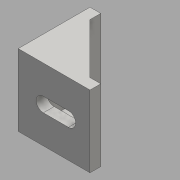
# Autodesk Inventor part: GUSSET 2020
Saved by Autodesk Inventor 2016 (Build 200138000, 138)
## iProperties
Created: 2023-12-31
Part Number: GUSSET 2020
Material: Generic
Document SubType Name: Modeling
Designer: Riskinova Oktavia
Density: 1 g/cm^3
Appearance: Default
Author: Riskinova Oktavia
Autodesk Inventor part; units mm, degrees
ref_plane "YZ Plane" through (0, 0, 0) normal (1, 0, 0) x (0, 1, 0)
ref_plane "XZ Plane" through (0, 0, 0) normal (0, 1, 0) x (-1, 0, 0)
ref_plane "XY Plane" through (0, 0, 0) normal (0, 0, 1) x (1, 0, 0)
sketch "Sketch1" plane through (0, 0, 0) normal (0, 0, 1) x (1, 0, 0)
  line L0 (0, 0) -> (0, 20)
  line L1 (0, 0) -> (20, 0)
  line L2 (0, 20) -> (3, 20)
  line L3 (3, 20) -> (3, 17)
  line L4 (3, 17) -> (17, 3)
  line L5 (17, 3) -> (20, 3)
  line L6 (20, 3) -> (20, 0)
  dimension "d0" = 20
  dimension "d1" = 20
  dimension "d2" = 3
  dimension "d3" = 3
  dimension "d4" = 3
  dimension "d5" = 3
  constraints: 14 end point, 2 horizontal, 2 vertical, 1 parallel, 1 perpendicular
  measures "d0" distance of L0.start L1.end
  measures "d1" distance of L0.start L0.end
  measures "d2" distance of L0.end L2.end
  measures "d3" distance of L5.end L1.end
  measures "d4" distance of L2.end L3.end
  measures "d5" distance of L4.end L5.end
extrude "Extrusion1" add sketch "Sketch1" along normal mid plane 20
sketch "Sketch2" plane through (0, 20, 10) normal (0, 1, 0) x (1, 0, 0)
  line L0 (3, 2) -> (17, 2)
  line L1 (17, 2) -> (17, 18)
  line L2 (17, 18) -> (3, 18)
  line L3 (3, 18) -> (3, 2)
  line L4 (0, 0) -> (0, 20) projected
  line L5 (3, 0) -> (3, 20) projected
  line L6 (17, 0) -> (17, 20) projected
  line L7 (3, 20) -> (17, 20) projected
  point P0 (0, 10)
  point P1 (3, 10)
  point P2 (0, 10)
  dimension "d8" = 2
  constraints: 8 end point, 2 collinear, 2 midpoint, 2 parallel, 1 horizontal, 1 horizontal alignment, 1 perpendicular
  measures "d8" distance between parallel lines of L7 L2
extrude "Extrusion2" cut sketch "Sketch2" against normal up to surface (17 mm away) contours L3 L2 L1 L0
sketch "Sketch3" plane through (17, 3, 10) normal (0, 1, 0) x (1, 0, 0)
  line L0 (-10, 10) -> (-3, 10) construction
  line L1 (-10, 8) -> (-3, 8)
  line L2 (-3, 12) -> (-10, 12)
  arc A0 (-10, 12) -> (-10, 8) centre (-10, 10) ccw
  arc A1 (-3, 8) -> (-3, 12) centre (-3, 10) ccw
  line L3 (-17, 0) -> (-17, 20) projected
  line L4 (-14, 0) -> (-14, 20) projected
  line L5 (3, 0) -> (3, 20) projected
  point P0 (-17, 10)
  point P1 (-6.5, 10)
  point P2 (-17, 10)
  point P3 (-17, 10)
  dimension "d11" = 4
  dimension "d12" = 4
  dimension "d21" = 6
  constraints: 8 end point, 4 point on circle, 4 tangent, 3 midpoint, 2 centre point, 1 horizontal, 1 horizontal alignment, 1 parallel
  measures "d11" distance between parallel lines of L2 L1
  measures "d12" distance from line of L0.start L4
  measures "d21" distance from line of L5 L0.end
extrude "Extrusion3" cut sketch "Sketch3" against normal through all
sketch "Sketch4" plane through (3, 17, 10) normal (1, 0, 0) x (0, 0, -1)
  line L0 (10, -3) -> (10, -10) construction
  line L1 (8, -3) -> (8, -10)
  line L2 (12, -10) -> (12, -3)
  arc A0 (12, -3) -> (8, -3) centre (10, -3) ccw
  arc A1 (8, -10) -> (12, -10) centre (10, -10) ccw
  line L3 (0, -17) -> (20, -17) projected
  line L4 (0, -14) -> (20, -14) projected
  line L5 (0, 3) -> (20, 3) projected
  point P0 (10, -17)
  point P1 (10, -6.5)
  point P2 (10, -17)
  dimension "d16" = 4
  dimension "d17" = 4
  dimension "d18" = 6
  constraints: 8 end point, 4 point on circle, 4 tangent, 2 centre point, 2 midpoint, 1 parallel, 1 vertical, 1 vertical alignment
  measures "d16" distance between parallel lines of L2 L1
  measures "d17" distance from line of L0.end L4
  measures "d18" distance from line of L0.start L5
extrude "Extrusion4" cut sketch "Sketch4" against normal through all
equation "\"d1\" = d0"
equation "\"d5\" = d2"
body "Solid1"
